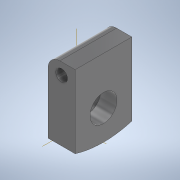
# Autodesk Inventor part: drag release plate
Saved by Autodesk Inventor 2021.1 (Build 251245000, 245)
## iProperties
Created: 2021-02-18
Part Number: drag release plate
Material: Generic
Document SubType Name: Modeling
Designer: Vamshi
Density: 1 g/cm^3
Appearance: Silicon Nitride - Polished
Author: Vamshi
Autodesk Inventor part; units mm, degrees
ref_plane "YZ Plane" through (0, 0, 0) normal (1, 0, 0) x (0, 1, 0)
ref_plane "XZ Plane" through (0, 0, 0) normal (0, 1, 0) x (-1, 0, 0)
ref_plane "XY Plane" through (0, 0, 0) normal (0, 0, 1) x (1, 0, 0)
sketch "Sketch1" plane through (0, 0, 0) normal (1, 0, 0) x (0, 1, 0)
  arc A0 (4.6958, 31.5) -> (4.6958, -31.5) centre (108, 0) ccw
  line L0 (4.6958, 31.5) -> (85.6007, 31.5)
  line L1 (85.6007, 31.5) -> (85.6007, -31.5)
  line L2 (85.6007, -31.5) -> (4.6958, -31.5)
  point P0 (0, 0)
  point P1 (0, 0)
  point P2 (4.6958, -31.5)
  dimension "d0" = 108
  dimension "d1" = 63
  dimension "d2" = 0
  constraints: 6 end point, 3 point on circle, 1 centre point, 1 coincident, 1 horizontal, 1 parallel, 1 perpendicular, 1 vertical alignment
  measures "d0" radius of A0
  measures "d1" distance of L0.end L1.end
  measures "d2" distance of A0.end L2.end
extrude "Extrusion1" add sketch "Sketch1" along normal blind 30
fillet "Fillet1" radius 13 1 edges at (0, 85.6007, 0)
sketch "Sketch2" plane through (0, 4.6958, 31.5) normal (0, 0, 1) x (1, 0, 0)
  circle A0 centre (15, 67.9049) radius 6.5
  line L0 (13, 80.9049) -> (30, 80.9049) projected
  line L1 (30, 80.9049) -> (30, 0) projected
  point P0 (0, -4.6958)
  dimension "d7" = 13
  dimension "d8" = 15
  dimension "d9" = 13
  constraints: 1 centre point
  measures "d7" distance from line of A0.centre L0
  measures "d8" distance from line of L1 A0.centre
  measures "d9" diameter of A0
extrude "Extrusion2" cut sketch "Sketch2" against normal through all
sketch "Sketch3" plane through (0, 0, 0) normal (-1, 0, 0) x (0, 0, 1)
  point P0 (0, 0)
  point P1 (0, 33)
  dimension "d12" = 33
  measures "d12" distance of point (0, 0) point (0, 33)
hole "Hole1" at (0, 33, 0) direction (1, 0, 0) diameter 30 end through all counterbore diameter 42 counterbore depth 12
body "Solid1"
